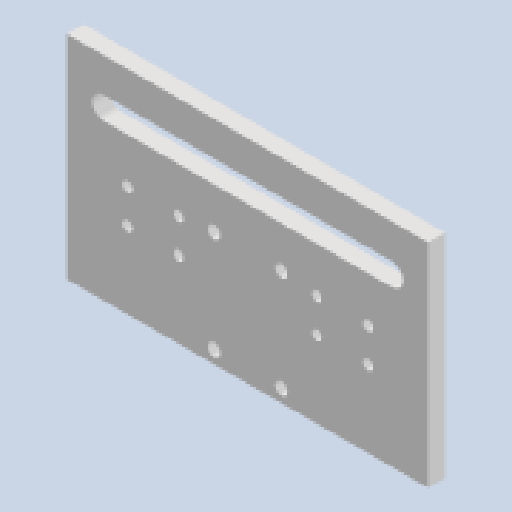
# Autodesk Inventor part: деталь на которой рельсы
Saved by Autodesk Inventor 2024.2 (Build 282272000, 272)
## iProperties
Created: 2025-11-27
Part Number: деталь на которой рельсы
Material: Типовые
Document SubType Name: Modeling
Designer: katya_notebook
Density: 1 g/cm^3
Appearance: По умолчанию
Author: katya_notebook
Autodesk Inventor part; units mm, degrees
ref_plane "YZ Plane" through (0, 0, 0) normal (1, 0, 0) x (0, 1, 0)
ref_plane "XZ Plane" through (0, 0, 0) normal (0, 1, 0) x (-1, 0, 0)
ref_plane "XY Plane" through (0, 0, 0) normal (0, 0, 1) x (1, 0, 0)
ref_plane "РабПлоскость1" through (30.6718, 18.7359, 5.7) normal (0, 0, 1) x (1, 0, 0)
sketch "Эскиз1" plane through (30.6718, 18.7359, 5.7) normal (0, 0, 1) x (1, 0, 0)
  line L0 (-3.7, 0) -> (-8.3, 0) projected
  line L1 (-8.3, 0) -> (-8.3, -13.5) projected
  line L2 (-3.7, -13.5) -> (-8.3, -13.5) projected
  line L3 (-3.7, -13.5) -> (-3.7, 0) projected
  circle A0 centre (-6, -2.75) radius 1.2 projected
  circle A1 centre (-6, -10.75) radius 1.2 projected
  line L4 (8.3, 0) -> (3.7, 0) projected
  line L5 (3.7, 0) -> (3.7, -13.5) projected
  line L6 (8.3, -13.5) -> (3.7, -13.5) projected
  line L7 (8.3, -13.5) -> (8.3, 0) projected
  circle A2 centre (6, -2.75) radius 1.2 projected
  circle A3 centre (6, -10.75) radius 1.2 projected
  line L8 (40.9, 0) -> (36.3, 0) projected
  line L9 (36.3, 0) -> (36.3, -13.5) projected
  line L10 (40.9, -13.5) -> (36.3, -13.5) projected
  line L11 (40.9, -13.5) -> (40.9, 0) projected
  circle A4 centre (38.6, -2.75) radius 1.2 projected
  circle A5 centre (38.6, -10.75) radius 1.2 projected
  line L12 (52.9, 0) -> (48.3, 0) projected
  line L13 (48.3, 0) -> (48.3, -13.5) projected
  line L14 (52.9, -13.5) -> (48.3, -13.5) projected
  line L15 (52.9, -13.5) -> (52.9, 0) projected
  circle A6 centre (50.6, -2.75) radius 1.2 projected
  circle A7 centre (50.6, -10.75) radius 1.2 projected
  circle A8 centre (-11.7, 10.5) radius 2.5 projected
  circle A9 centre (-11.7, 10.5) radius 1 projected
  circle A10 centre (16.3, -17.5) radius 2.5 projected
  circle A11 centre (16.3, -17.5) radius 1 projected
  line L16 (-20.2279, 21.2173) -> (64.7721, 21.2173)
  line L17 (64.7721, 21.2173) -> (64.7721, -28.7827)
  line L18 (64.7721, -28.7827) -> (-20.2279, -28.7827)
  line L19 (-20.2279, -28.7827) -> (-20.2279, 21.2173)
  line L20 (22.2721, -16.5) -> (22.2721, -5.5248)
  line L21 (13.8, -23.7827) -> (31.824, -23.7827)
  circle A12 centre (-11.7, 10.5) radius 2.65
  line L22 (-11.7, 13.15) -> (56.2443, 13.15)
  line L23 (-11.7, 7.85) -> (56.2443, 7.85)
  circle A13 centre (56.2443, 10.5) radius 2.65
  point P0 (-30.6718, -18.7359)
  point P1 (-20.2279, -3.7827)
  dimension "d0" = 50
  dimension "d1" = 85
  dimension "d2" = 42.5
  dimension "d3" = 5
  dimension "d4" = 5.3
  constraints: 16 end point, 5 horizontal, 4 point on circle, 2 centre point, 2 parallel, 2 tangent, 2 vertical, 1 coincident, 1 midpoint, 1 perpendicular, 1 symmetric about line, 1 other
  measures "d0" distance of L16.end L17.end
  measures "d1" distance of L16.start L16.end
  measures "d2" distance from line of point (-20.228, -3.783) L20
  measures "d3" distance between parallel lines of L18 L21
  measures "d4" diameter of A12
extrude "Выдавливание1" add sketch "Эскиз1" along normal blind 4 contours L3 L2 L1 L0 | L7 L6 L5 L4 | L11 L10 L9 L8 | L15 L14 L13 L12 | A10 | A11 | L16 L17 L18 L19
sketch "Эскиз2" plane through (30.6718, 18.7359, 9.7) normal (0, 0, 1) x (1, 0, 0)
  circle A0 centre (14.35, -1.7827) radius 1.5 projected
  circle A1 centre (30.25, -1.7827) radius 1.5 projected
  circle A2 centre (14.35, -25.7827) radius 1.5 projected
  circle A3 centre (30.25, -25.7827) radius 1.5 projected
  point P0 (-30.6718, -18.7359)
extrude "Выдавливание2" cut sketch "Эскиз2" against normal blind 10
